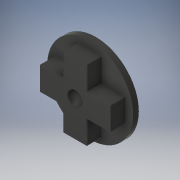
# Autodesk Inventor part: DPAD-Gameboy
Saved by Autodesk Inventor 2019 (Build 230136000, 136)
## iProperties
Created: 2019-04-18
Part Number: DPAD-Gameboy
Material: Plastique ABS
Document SubType Name: Modeling
Designer: Sébastien DI MERCURIO
Density: 1.06 g/cm^3
Appearance: Lisse - Noir
Author: Sébastien DI MERCURIO
Autodesk Inventor part; units mm, degrees
ref_plane "YZ Plane" through (0, 0, 0) normal (1, 0, 0) x (0, 1, 0)
ref_plane "XZ Plane" through (0, 0, 0) normal (0, 1, 0) x (-1, 0, 0)
ref_plane "XY Plane" through (0, 0, 0) normal (0, 0, 1) x (1, 0, 0)
sketch "Esquisse1" plane through (0, 0, 0) normal (0, 0, 1) x (1, 0, 0)
  circle A0 centre (0, 0) radius 12.75
  dimension "d0" = 25.5
  constraints: 1 centre point, 1 coincident
  measures "d0" diameter of A0
extrude "Extrusion1" add sketch "Esquisse1" along normal blind 1.7
sketch "Esquisse2" plane through (0, 0, 1.7) normal (0, 0, 1) x (1, 0, 0)
  line L0 (-3.5, 10.5) -> (3.5, 10.5)
  line L1 (3.5, 10.5) -> (3.5, -10.5)
  line L2 (3.5, -10.5) -> (-3.5, -10.5)
  line L3 (-3.5, -10.5) -> (-3.5, 10.5)
  line L4 (-10.5, 3.5) -> (10.5, 3.5)
  line L5 (10.5, 3.5) -> (10.5, -3.5)
  line L6 (10.5, -3.5) -> (-10.5, -3.5)
  line L7 (-10.5, -3.5) -> (-10.5, 3.5)
  point P0 (0, 0)
  dimension "d3" = 7
  dimension "d4" = 7
  dimension "d5" = 3.5
  dimension "d6" = 3.5
  dimension "d7" = 21
  dimension "d8" = 21
  dimension "d9" = 10.5
  dimension "d10" = 10.5
  constraints: 16 end point, 4 parallel, 2 horizontal, 2 perpendicular
  measures "d3" distance of L0.start L0.end
  measures "d4" distance of L6.end L4.start
  measures "d5" horizontal distance of point (0, 0) L0.start
  measures "d6" vertical distance of point (0, 0) L4.start
  measures "d7" distance between parallel lines of L5 L7
  measures "d8" distance between parallel lines of L2 L0
  measures "d9" horizontal distance of point (0, 0) L4.start
  measures "d10" vertical distance of point (0, 0) L0.end
extrude "Extrusion2" add sketch "Esquisse2" along normal blind 4.5
sketch "Esquisse3" plane through (0, 0, 0) normal (0, 0, -1) x (-1, 0, 0)
  line L0 (-1.25, 9) -> (1.25, 9)
  line L1 (1.25, 9) -> (1.25, -9)
  line L2 (1.25, -9) -> (-1.25, -9)
  line L3 (-1.25, -9) -> (-1.25, 9)
  line L4 (-9, 1.25) -> (9, 1.25)
  line L5 (9, 1.25) -> (9, -1.25)
  line L6 (9, -1.25) -> (-9, -1.25)
  line L7 (-9, -1.25) -> (-9, 1.25)
  point P0 (0, 0)
  dimension "d13" = 2.5
  dimension "d14" = 2.5
  dimension "d15" = 1.25
  dimension "d16" = 1.25
  dimension "d17" = 18
  dimension "d18" = 18
  dimension "d19" = 9
  dimension "d20" = 9
  constraints: 16 end point, 4 parallel, 2 horizontal, 2 perpendicular
  measures "d13" distance between parallel lines of L1 L3
  measures "d14" distance of L6.end L4.start
  measures "d15" vertical distance of point (0, 0) L4.start
  measures "d16" horizontal distance of point (0, 0) L0.start
  measures "d17" distance between parallel lines of L2 L0
  measures "d18" distance between parallel lines of L5 L7
  measures "d19" horizontal distance of point (0, 0) L4.start
  measures "d20" vertical distance of point (0, 0) L0.end
extrude "Extrusion3" cut sketch "Esquisse3" against normal blind 4
sketch "Esquisse4" plane through (0, 0, 4) normal (0, 0, -1) x (-1, 0, 0)
  circle A0 centre (0, 0) radius 2.9
  dimension "d23" = 5.8
  constraints: 1 centre point, 1 coincident
  measures "d23" diameter of A0
extrude "Extrusion4" add sketch "Esquisse4" along normal blind 6.7
fillet "Congé1" radius 2.9 1 edges at (2.9, 0, -2.7)
sketch "Esquisse5" plane through (0, 0, 6.2) normal (0, 0, 1) x (1, 0, 0)
  circle A0 centre (0, 0) radius 2.25
  dimension "d27" = 4.5
  constraints: 1 centre point, 1 coincident
  measures "d27" diameter of A0
extrude "Extrusion5" cut sketch "Esquisse5" against normal blind 2.25
fillet "Congé2" radius 2.25 1 edges at (-2.25, 0, 3.95)
fillet "Congé3" radius 0.1 20 edges at (-3.5, 7, 6.2) (0, 10.5, 6.2) (3.5, 7, 6.2) (7, 3.5, 6.2) (10.5, 0, 6.2) (7, -3.5, 6.2) (3.5, -7, 6.2) (0, -10.5, 6.2) (-3.5, -7, 6.2) (-7, -3.5, 6.2) (-10.5, 0, 6.2) (-7, 3.5, 6.2) (-3.5, 10.5, 3.95) (-10.5, 3.5, 3.95) (-10.5, -3.5, 3.95) (-3.5, -10.5, 3.95) (3.5, -10.5, 3.95) (10.5, -3.5, 3.95) (10.5, 3.5, 3.95) (3.5, 10.5, 3.95)
equation "\"d4\" = d3"
equation "\"d5\" = 0.5 * d3"
equation "\"d6\" = 0.5 * d4"
equation "\"d8\" = d7"
equation "\"d9\" = 0.5 * d7"
equation "\"d10\" = 0.5 * d7"
equation "\"d14\" = d13"
equation "\"d15\" = 0.5 * d13"
equation "\"d16\" = 0.5 * d13"
equation "\"d18\" = d17"
equation "\"d19\" = 0.5 * d17"
equation "\"d20\" = 0.5 * d17"
